Autodesk Inventor part; units mm, degrees
(part 2 of 2)
sketch "Esboço25" plane through (-2.4, 91.8, 35) normal (0, 1, 0) x (1, 0, 0)
  line L0 (50.4433, 30.11) -> (47.6201, 28.48)
  line L1 (50.4433, 33.37) -> (50.4433, 30.11)
  line L2 (47.6201, 28.48) -> (44.7968, 30.11)
  line L3 (44.7968, 30.11) -> (44.7968, 33.37)
  line L4 (47.6201, 35) -> (50.4433, 33.37)
  line L5 (44.7968, 33.37) -> (47.6201, 35)
  line L6 (47.6201, 28.48) -> (47.6201, 27.48)
  line L7 (50.4433, 22.59) -> (47.6201, 20.96)
  line L8 (50.4433, 25.85) -> (50.4433, 22.59)
  line L9 (47.6201, 20.96) -> (44.7968, 22.59)
  line L10 (44.7968, 22.59) -> (44.7968, 25.85)
  line L11 (47.6201, 27.48) -> (50.4433, 25.85)
  line L12 (44.7968, 25.85) -> (47.6201, 27.48)
  line L13 (47.6201, 20.96) -> (47.6201, 19.96)
  line L14 (50.4433, 15.07) -> (47.6201, 13.44)
  line L15 (50.4433, 18.33) -> (50.4433, 15.07)
  line L16 (47.6201, 13.44) -> (44.7968, 15.07)
  line L17 (44.7968, 15.07) -> (44.7968, 18.33)
  line L18 (47.6201, 19.96) -> (50.4433, 18.33)
  line L19 (44.7968, 18.33) -> (47.6201, 19.96)
  line L20 (47.6201, 13.44) -> (47.6201, 12.44)
  line L21 (50.4433, 7.55) -> (47.6201, 5.92)
  line L22 (50.4433, 10.81) -> (50.4433, 7.55)
  line L23 (47.6201, 5.92) -> (44.7968, 7.55)
  line L24 (44.7968, 7.55) -> (44.7968, 10.81)
  line L25 (47.6201, 12.44) -> (50.4433, 10.81)
  line L26 (44.7968, 10.81) -> (47.6201, 12.44)
  line L27 (47.6201, 5.92) -> (47.6201, 4.92)
  line L28 (47.6201, 1) -> (47.6201, 4.92)
  line L29 (47.6201, 1) -> (45.9227, 1.98)
  line L30 (45.9227, 1.98) -> (45.9227, 3.94)
  line L31 (45.9227, 3.94) -> (47.6201, 4.92)
  line L32 (47.6201, 4.92) -> (49.3175, 3.94)
  line L33 (49.3175, 3.94) -> (49.3175, 1.98)
  line L34 (49.3175, 1.98) -> (47.6201, 1)
  line L35 (39.9968, 30.11) -> (37.1736, 28.48)
  line L36 (39.9968, 33.37) -> (39.9968, 30.11)
  line L37 (37.1736, 28.48) -> (34.3504, 30.11)
  line L38 (34.3504, 30.11) -> (34.3504, 33.37)
  line L39 (37.1736, 35) -> (39.9968, 33.37)
  line L40 (34.3504, 33.37) -> (37.1736, 35)
  line L41 (37.1736, 28.48) -> (37.1736, 27.48)
  line L42 (37.1736, 20.96) -> (37.1736, 19.96)
  line L43 (39.9968, 22.59) -> (37.1736, 20.96)
  line L44 (37.1736, 20.96) -> (34.3504, 22.59)
  line L45 (39.9968, 25.85) -> (39.9968, 22.59)
  line L46 (34.3504, 22.59) -> (34.3504, 25.85)
  line L47 (37.1736, 27.48) -> (39.9968, 25.85)
  line L48 (34.3504, 25.85) -> (37.1736, 27.48)
  line L49 (37.1736, 13.44) -> (37.1736, 12.44)
  line L50 (39.9968, 15.07) -> (37.1736, 13.44)
  line L51 (37.1736, 13.44) -> (34.3504, 15.07)
  line L52 (39.9968, 18.33) -> (39.9968, 15.07)
  line L53 (34.3504, 15.07) -> (34.3504, 18.33)
  line L54 (37.1736, 19.96) -> (39.9968, 18.33)
  line L55 (34.3504, 18.33) -> (37.1736, 19.96)
  line L56 (37.1736, 5.92) -> (37.1736, 4.92)
  line L57 (39.9968, 7.55) -> (37.1736, 5.92)
  line L58 (37.1736, 5.92) -> (34.3504, 7.55)
  line L59 (39.9968, 10.81) -> (39.9968, 7.55)
  line L60 (34.3504, 7.55) -> (34.3504, 10.81)
  line L61 (37.1736, 12.44) -> (39.9968, 10.81)
  line L62 (34.3504, 10.81) -> (37.1736, 12.44)
  line L63 (37.1736, 1) -> (37.1736, 4.92)
  line L64 (37.1736, 1) -> (35.4762, 1.98)
  line L65 (35.4762, 1.98) -> (35.4762, 3.94)
  line L66 (35.4762, 3.94) -> (37.1736, 4.92)
  line L67 (37.1736, 4.92) -> (38.871, 3.94)
  line L68 (38.871, 3.94) -> (38.871, 1.98)
  line L69 (38.871, 1.98) -> (37.1736, 1)
  line L70 (29.5504, 30.11) -> (26.7271, 28.48)
  line L71 (29.5504, 33.37) -> (29.5504, 30.11)
  line L72 (26.7271, 28.48) -> (23.9039, 30.11)
  line L73 (23.9039, 30.11) -> (23.9039, 33.37)
  line L74 (26.7271, 35) -> (29.5504, 33.37)
  line L75 (23.9039, 33.37) -> (26.7271, 35)
  line L76 (26.7271, 28.48) -> (26.7271, 27.48)
  line L77 (26.7271, 20.96) -> (26.7271, 19.96)
  line L78 (29.5504, 22.59) -> (26.7271, 20.96)
  line L79 (26.7271, 20.96) -> (23.9039, 22.59)
  line L80 (29.5504, 25.85) -> (29.5504, 22.59)
  line L81 (23.9039, 22.59) -> (23.9039, 25.85)
  line L82 (26.7271, 27.48) -> (29.5504, 25.85)
  line L83 (23.9039, 25.85) -> (26.7271, 27.48)
  line L84 (26.7271, 13.44) -> (26.7271, 12.44)
  line L85 (29.5504, 15.07) -> (26.7271, 13.44)
  line L86 (26.7271, 13.44) -> (23.9039, 15.07)
  line L87 (29.5504, 18.33) -> (29.5504, 15.07)
  line L88 (23.9039, 15.07) -> (23.9039, 18.33)
  line L89 (26.7271, 19.96) -> (29.5504, 18.33)
  line L90 (23.9039, 18.33) -> (26.7271, 19.96)
  line L91 (26.8228, 5.92) -> (26.8228, 4.7542)
  line L92 (29.5504, 7.55) -> (26.7271, 5.92)
  line L93 (26.7271, 5.92) -> (23.9039, 7.55)
  line L94 (29.5504, 10.81) -> (29.5504, 7.55)
  line L95 (23.9039, 7.55) -> (23.9039, 10.81)
  line L96 (26.7271, 12.44) -> (29.5504, 10.81)
  line L97 (23.9039, 10.81) -> (26.7271, 12.44)
  line L98 (26.8228, 1.0553) -> (26.8228, 4.7542)
  line L99 (26.8228, 1.0553) -> (25.2211, 1.98)
  line L100 (25.2211, 1.98) -> (25.2211, 3.8295)
  line L101 (25.2211, 3.8295) -> (26.8228, 4.7542)
  line L102 (26.8228, 4.7542) -> (28.4245, 3.8295)
  line L103 (28.4245, 3.8295) -> (28.4245, 1.98)
  line L104 (28.4245, 1.98) -> (26.8228, 1.0553)
  line L105 (19.1039, 30.11) -> (16.2806, 28.48)
  line L106 (19.1039, 33.37) -> (19.1039, 30.11)
  line L107 (16.2806, 28.48) -> (13.4574, 30.11)
  line L108 (13.4574, 30.11) -> (13.4574, 33.37)
  line L109 (16.2806, 35) -> (19.1039, 33.37)
  line L110 (13.4574, 33.37) -> (16.2806, 35)
  line L111 (16.2806, 28.48) -> (16.2806, 27.48)
  line L112 (16.2806, 20.96) -> (16.2806, 19.96)
  line L113 (19.1039, 22.59) -> (16.2806, 20.96)
  line L114 (16.2806, 20.96) -> (13.4574, 22.59)
  line L115 (19.1039, 25.85) -> (19.1039, 22.59)
  line L116 (13.4574, 22.59) -> (13.4574, 25.85)
  line L117 (16.2806, 27.48) -> (19.1039, 25.85)
  line L118 (13.4574, 25.85) -> (16.2806, 27.48)
  line L119 (16.2806, 13.44) -> (16.2806, 12.44)
  line L120 (19.1039, 15.07) -> (16.2806, 13.44)
  line L121 (16.2806, 13.44) -> (13.4574, 15.07)
  line L122 (19.1039, 18.33) -> (19.1039, 15.07)
  line L123 (13.4574, 15.07) -> (13.4574, 18.33)
  line L124 (16.2806, 19.96) -> (19.1039, 18.33)
  line L125 (13.4574, 18.33) -> (16.2806, 19.96)
  line L126 (16.2806, 5.92) -> (16.2806, 4.92)
  line L127 (19.1039, 7.55) -> (16.2806, 5.92)
  line L128 (16.2806, 5.92) -> (13.4574, 7.55)
  line L129 (19.1039, 10.81) -> (19.1039, 7.55)
  line L130 (13.4574, 7.55) -> (13.4574, 10.81)
  line L131 (16.2806, 12.44) -> (19.1039, 10.81)
  line L132 (13.4574, 10.81) -> (16.2806, 12.44)
  line L133 (16.2806, 1) -> (16.2806, 4.92)
  line L134 (16.2806, 1) -> (14.5832, 1.98)
  line L135 (14.5832, 1.98) -> (14.5832, 3.94)
  line L136 (14.5832, 3.94) -> (16.2806, 4.92)
  line L137 (16.2806, 4.92) -> (17.978, 3.94)
  line L138 (17.978, 3.94) -> (17.978, 1.98)
  line L139 (17.978, 1.98) -> (16.2806, 1)
  line L140 (8.6574, 30.11) -> (5.8342, 28.48)
  line L141 (8.6574, 33.37) -> (8.6574, 30.11)
  line L142 (5.8342, 28.48) -> (3.0109, 30.11)
  line L143 (3.0109, 30.11) -> (3.0109, 33.37)
  line L144 (5.8342, 35) -> (8.6574, 33.37)
  line L145 (3.0109, 33.37) -> (5.8342, 35)
  line L146 (5.8342, 28.48) -> (5.8342, 27.48)
  line L147 (5.8342, 20.96) -> (5.8342, 19.96)
  line L148 (8.6574, 22.59) -> (5.8342, 20.96)
  line L149 (5.8342, 20.96) -> (3.0109, 22.59)
  line L150 (8.6574, 25.85) -> (8.6574, 22.59)
  line L151 (3.0109, 22.59) -> (3.0109, 25.85)
  line L152 (5.8342, 27.48) -> (8.6574, 25.85)
  line L153 (3.0109, 25.85) -> (5.8342, 27.48)
  line L154 (5.8342, 13.44) -> (5.8342, 12.44)
  line L155 (8.6574, 15.07) -> (5.8342, 13.44)
  line L156 (5.8342, 13.44) -> (3.0109, 15.07)
  line L157 (8.6574, 18.33) -> (8.6574, 15.07)
  line L158 (3.0109, 15.07) -> (3.0109, 18.33)
  line L159 (5.8342, 19.96) -> (8.6574, 18.33)
  line L160 (3.0109, 18.33) -> (5.8342, 19.96)
  line L161 (5.8769, 5.92) -> (5.8769, 4.8459)
  line L162 (8.6574, 7.55) -> (5.8342, 5.92)
  line L163 (5.8342, 5.92) -> (3.0109, 7.55)
  line L164 (8.6574, 10.81) -> (8.6574, 7.55)
  line L165 (3.0109, 7.55) -> (3.0109, 10.81)
  line L166 (5.8342, 12.44) -> (8.6574, 10.81)
  line L167 (3.0109, 10.81) -> (5.8342, 12.44)
  line L168 (5.8769, 1.0247) -> (5.8769, 4.8459)
  line L169 (5.8769, 1.0247) -> (4.2223, 1.98)
  line L170 (4.2223, 1.98) -> (4.2223, 3.8906)
  line L171 (4.2223, 3.8906) -> (5.8769, 4.8459)
  line L172 (5.8769, 4.8459) -> (7.5316, 3.8906)
  line L173 (7.5316, 3.8906) -> (7.5316, 1.98)
  line L174 (7.5316, 1.98) -> (5.8769, 1.0247)
  line L175 (3.0109, 9.18) -> (3.0109, 7.7242)
  line L176 (60.8898, 7.55) -> (58.0666, 5.92)
  line L177 (58.0666, 5.92) -> (55.2433, 7.55)
  line L178 (60.8898, 10.81) -> (60.8898, 7.55)
  line L179 (55.2433, 7.55) -> (55.2433, 10.81)
  line L180 (58.0666, 12.44) -> (60.8898, 10.81)
  line L181 (55.2433, 10.81) -> (58.0666, 12.44)
  line L182 (58.0666, 1) -> (56.3692, 1.98)
  line L183 (56.3692, 1.98) -> (56.3692, 3.94)
  line L184 (56.3692, 3.94) -> (58.0666, 4.92)
  line L185 (58.0666, 4.92) -> (59.764, 3.94)
  line L186 (59.764, 3.94) -> (59.764, 1.98)
  line L187 (59.764, 1.98) -> (58.0666, 1)
  line L188 (60.8898, 30.11) -> (58.0666, 28.48)
  line L189 (60.8898, 33.37) -> (60.8898, 30.11)
  line L190 (58.0666, 28.48) -> (55.2433, 30.11)
  line L191 (55.2433, 30.11) -> (55.2433, 33.37)
  line L192 (58.0666, 35) -> (60.8898, 33.37)
  line L193 (55.2433, 33.37) -> (58.0666, 35)
  line L194 (5.8342, 7.5447) -> (8.6574, 5.9147)
  line L195 (3.0109, 5.9147) -> (5.8342, 7.5447)
  line L196 (8.6574, 5.9147) -> (8.6574, 2.6547)
  line L197 (8.6574, 2.6547) -> (5.8342, 1.0247)
  line L198 (3.0109, 2.6547) -> (3.0109, 5.9147)
  line L199 (5.8342, 1.0247) -> (3.0109, 2.6547)
  line L200 (8.6574, 33.37) -> (8.6574, 2.6547)
  line L201 (3.0109, 33.37) -> (3.0109, 2.6547)
  line L202 (19.1039, 30.11) -> (16.2806, 28.48)
  line L203 (16.2806, 28.48) -> (13.4574, 30.11)
  line L204 (19.1039, 33.37) -> (19.1039, 30.11)
  line L205 (13.4574, 30.11) -> (13.4574, 33.37)
  line L206 (16.2806, 28.48) -> (16.2806, 27.48)
  line L207 (16.2806, 27.48) -> (19.1039, 25.85)
  line L208 (13.4574, 25.85) -> (16.2806, 27.48)
  line L209 (19.1039, 25.85) -> (19.1039, 22.59)
  line L210 (13.4574, 22.59) -> (13.4574, 25.85)
  line L211 (16.2806, 20.96) -> (13.4574, 22.59)
  line L212 (16.2806, 20.96) -> (16.2806, 19.96)
  line L213 (19.1039, 22.59) -> (16.2806, 20.96)
  line L214 (16.2806, 19.96) -> (19.1039, 18.33)
  line L215 (13.4574, 18.33) -> (16.2806, 19.96)
  line L216 (19.1039, 18.33) -> (19.1039, 15.07)
  line L217 (13.4574, 15.07) -> (13.4574, 18.33)
  line L218 (16.2806, 13.44) -> (13.4574, 15.07)
  line L219 (19.1039, 15.07) -> (16.2806, 13.44)
  line L220 (16.2806, 13.44) -> (16.2806, 12.44)
  line L221 (16.2806, 12.44) -> (19.1039, 10.81)
  line L222 (13.4574, 10.81) -> (16.2806, 12.44)
  line L223 (19.1039, 10.81) -> (19.1039, 7.55)
  line L224 (19.1039, 7.55) -> (16.2806, 5.92)
  line L225 (13.4574, 7.55) -> (13.4574, 10.81)
  line L226 (16.2806, 5.92) -> (13.4574, 7.55)
  line L227 (16.3234, 5.92) -> (16.3234, 4.8459)
  line L228 (14.6687, 3.8906) -> (16.3234, 4.8459)
  line L229 (16.3234, 4.8459) -> (17.978, 3.8906)
  line L230 (17.978, 3.8906) -> (17.978, 1.98)
  line L231 (14.6687, 1.98) -> (14.6687, 3.8906)
  line L232 (16.3234, 1.0247) -> (16.3234, 4.8459)
  line L233 (17.978, 1.98) -> (16.3234, 1.0247)
  line L234 (16.3234, 1.0247) -> (14.6687, 1.98)
  line L235 (16.2806, 35) -> (19.1039, 33.37)
  line L236 (13.4574, 33.37) -> (16.2806, 35)
  line L237 (13.4574, 9.18) -> (13.4574, 7.7242)
  line L238 (13.4574, 5.9147) -> (16.2806, 7.5447)
  line L239 (13.4574, 2.6547) -> (13.4574, 5.9147)
  line L240 (16.2806, 1.0247) -> (13.4574, 2.6547)
  line L241 (19.1039, 2.6547) -> (16.2806, 1.0247)
  line L242 (19.1039, 5.9147) -> (19.1039, 2.6547)
  line L243 (16.2806, 7.5447) -> (19.1039, 5.9147)
  line L244 (19.1039, 33.37) -> (19.1039, 2.6547)
  line L245 (13.4574, 33.37) -> (13.4574, 2.6547)
  line L246 (29.5504, 30.11) -> (26.7271, 28.48)
  line L247 (26.7271, 28.48) -> (23.9039, 30.11)
  line L248 (29.5504, 33.37) -> (29.5504, 30.11)
  line L249 (23.9039, 30.11) -> (23.9039, 33.37)
  line L250 (26.7271, 28.48) -> (26.7271, 27.48)
  line L251 (26.7271, 27.48) -> (29.5504, 25.85)
  line L252 (23.9039, 25.85) -> (26.7271, 27.48)
  line L253 (29.5504, 25.85) -> (29.5504, 22.59)
  line L254 (23.9039, 22.59) -> (23.9039, 25.85)
  line L255 (26.7271, 20.96) -> (23.9039, 22.59)
  line L256 (26.7271, 20.96) -> (26.7271, 19.96)
  line L257 (29.5504, 22.59) -> (26.7271, 20.96)
  line L258 (26.7271, 19.96) -> (29.5504, 18.33)
  line L259 (23.9039, 18.33) -> (26.7271, 19.96)
  line L260 (29.5504, 18.33) -> (29.5504, 15.07)
  line L261 (23.9039, 15.07) -> (23.9039, 18.33)
  line L262 (26.7271, 13.44) -> (23.9039, 15.07)
  line L263 (29.5504, 15.07) -> (26.7271, 13.44)
  line L264 (26.7271, 13.44) -> (26.7271, 12.44)
  line L265 (26.7271, 12.44) -> (29.5504, 10.81)
  line L266 (23.9039, 10.81) -> (26.7271, 12.44)
  line L267 (29.5504, 10.81) -> (29.5504, 7.55)
  line L268 (29.5504, 7.55) -> (26.7271, 5.92)
  line L269 (23.9039, 7.55) -> (23.9039, 10.81)
  line L270 (26.7271, 5.92) -> (23.9039, 7.55)
  line L271 (26.7699, 5.92) -> (26.7699, 4.8459)
  line L272 (25.1152, 3.8906) -> (26.7699, 4.8459)
  line L273 (26.7699, 4.8459) -> (28.4245, 3.8906)
  line L274 (28.4245, 3.8906) -> (28.4245, 1.98)
  line L275 (25.1152, 1.98) -> (25.1152, 3.8906)
  line L276 (26.7699, 1.0247) -> (26.7699, 4.8459)
  line L277 (28.4245, 1.98) -> (26.7699, 1.0247)
  line L278 (26.7699, 1.0247) -> (25.1152, 1.98)
  line L279 (26.7271, 35) -> (29.5504, 33.37)
  line L280 (23.9039, 33.37) -> (26.7271, 35)
  line L281 (23.9039, 9.18) -> (23.9039, 7.7242)
  line L282 (23.9039, 5.9147) -> (26.7271, 7.5447)
  line L283 (23.9039, 2.6547) -> (23.9039, 5.9147)
  line L284 (26.7271, 1.0247) -> (23.9039, 2.6547)
  line L285 (29.5504, 2.6547) -> (26.7271, 1.0247)
  line L286 (29.5504, 5.9147) -> (29.5504, 2.6547)
  line L287 (26.7271, 7.5447) -> (29.5504, 5.9147)
  line L288 (29.5504, 33.37) -> (29.5504, 2.6547)
  line L289 (23.9039, 33.37) -> (23.9039, 2.6547)
  line L290 (39.9968, 30.11) -> (37.1736, 28.48)
  line L291 (37.1736, 28.48) -> (34.3504, 30.11)
  line L292 (39.9968, 33.37) -> (39.9968, 30.11)
  line L293 (34.3504, 30.11) -> (34.3504, 33.37)
  line L294 (37.1736, 28.48) -> (37.1736, 27.48)
  line L295 (37.1736, 27.48) -> (39.9968, 25.85)
  line L296 (34.3504, 25.85) -> (37.1736, 27.48)
  line L297 (39.9968, 25.85) -> (39.9968, 22.59)
  line L298 (34.3504, 22.59) -> (34.3504, 25.85)
  line L299 (37.1736, 20.96) -> (34.3504, 22.59)
  line L300 (37.1736, 20.96) -> (37.1736, 19.96)
  line L301 (39.9968, 22.59) -> (37.1736, 20.96)
  line L302 (37.1736, 19.96) -> (39.9968, 18.33)
  line L303 (34.3504, 18.33) -> (37.1736, 19.96)
  line L304 (39.9968, 18.33) -> (39.9968, 15.07)
  line L305 (34.3504, 15.07) -> (34.3504, 18.33)
  line L306 (37.1736, 13.44) -> (34.3504, 15.07)
  line L307 (39.9968, 15.07) -> (37.1736, 13.44)
  line L308 (37.1736, 13.44) -> (37.1736, 12.44)
  line L309 (37.1736, 12.44) -> (39.9968, 10.81)
  line L310 (34.3504, 10.81) -> (37.1736, 12.44)
  line L311 (39.9968, 10.81) -> (39.9968, 7.55)
  line L312 (39.9968, 7.55) -> (37.1736, 5.92)
  line L313 (34.3504, 7.55) -> (34.3504, 10.81)
  line L314 (37.1736, 5.92) -> (34.3504, 7.55)
  line L315 (37.2164, 5.92) -> (37.2164, 4.8459)
  line L316 (35.5617, 3.8906) -> (37.2164, 4.8459)
  line L317 (37.2164, 4.8459) -> (38.871, 3.8906)
  line L318 (38.871, 3.8906) -> (38.871, 1.98)
  line L319 (35.5617, 1.98) -> (35.5617, 3.8906)
  line L320 (37.2164, 1.0247) -> (37.2164, 4.8459)
  line L321 (38.871, 1.98) -> (37.2164, 1.0247)
  line L322 (37.2164, 1.0247) -> (35.5617, 1.98)
  line L323 (37.1736, 35) -> (39.9968, 33.37)
  line L324 (34.3504, 33.37) -> (37.1736, 35)
  line L325 (34.3504, 9.18) -> (34.3504, 7.7242)
  line L326 (34.3504, 5.9147) -> (37.1736, 7.5447)
  line L327 (34.3504, 2.6547) -> (34.3504, 5.9147)
  line L328 (37.1736, 1.0247) -> (34.3504, 2.6547)
  line L329 (39.9968, 2.6547) -> (37.1736, 1.0247)
  line L330 (39.9968, 5.9147) -> (39.9968, 2.6547)
  line L331 (37.1736, 7.5447) -> (39.9968, 5.9147)
  line L332 (39.9968, 33.37) -> (39.9968, 2.6547)
  line L333 (34.3504, 33.37) -> (34.3504, 2.6547)
  line L334 (50.4433, 30.11) -> (47.6201, 28.48)
  line L335 (47.6201, 28.48) -> (44.7968, 30.11)
  line L336 (50.4433, 33.37) -> (50.4433, 30.11)
  line L337 (44.7968, 30.11) -> (44.7968, 33.37)
  line L338 (47.6201, 28.48) -> (47.6201, 27.48)
  line L339 (47.6201, 27.48) -> (50.4433, 25.85)
  line L340 (44.7968, 25.85) -> (47.6201, 27.48)
  line L341 (50.4433, 25.85) -> (50.4433, 22.59)
  line L342 (44.7968, 22.59) -> (44.7968, 25.85)
  line L343 (47.6201, 20.96) -> (44.7968, 22.59)
  line L344 (47.6201, 20.96) -> (47.6201, 19.96)
  line L345 (50.4433, 22.59) -> (47.6201, 20.96)
  line L346 (47.6201, 19.96) -> (50.4433, 18.33)
  line L347 (44.7968, 18.33) -> (47.6201, 19.96)
  line L348 (50.4433, 18.33) -> (50.4433, 15.07)
  line L349 (44.7968, 15.07) -> (44.7968, 18.33)
  line L350 (47.6201, 13.44) -> (44.7968, 15.07)
  line L351 (50.4433, 15.07) -> (47.6201, 13.44)
  line L352 (47.6201, 13.44) -> (47.6201, 12.44)
  line L353 (47.6201, 12.44) -> (50.4433, 10.81)
  line L354 (44.7968, 10.81) -> (47.6201, 12.44)
  line L355 (50.4433, 10.81) -> (50.4433, 7.55)
  line L356 (50.4433, 7.55) -> (47.6201, 5.92)
  line L357 (44.7968, 7.55) -> (44.7968, 10.81)
  line L358 (47.6201, 5.92) -> (44.7968, 7.55)
  line L359 (47.6628, 5.92) -> (47.6628, 4.8459)
  line L360 (46.0082, 3.8906) -> (47.6628, 4.8459)
  line L361 (47.6628, 4.8459) -> (49.3175, 3.8906)
  line L362 (49.3175, 3.8906) -> (49.3175, 1.98)
  line L363 (46.0082, 1.98) -> (46.0082, 3.8906)
  line L364 (47.6628, 1.0247) -> (47.6628, 4.8459)
  line L365 (49.3175, 1.98) -> (47.6628, 1.0247)
  line L366 (47.6628, 1.0247) -> (46.0082, 1.98)
  line L367 (47.6201, 35) -> (50.4433, 33.37)
  line L368 (44.7968, 33.37) -> (47.6201, 35)
  line L369 (44.7968, 9.18) -> (44.7968, 7.7242)
  line L370 (44.7968, 5.9147) -> (47.6201, 7.5447)
  line L371 (44.7968, 2.6547) -> (44.7968, 5.9147)
  line L372 (47.6201, 1.0247) -> (44.7968, 2.6547)
  line L373 (50.4433, 2.6547) -> (47.6201, 1.0247)
  line L374 (50.4433, 5.9147) -> (50.4433, 2.6547)
  line L375 (47.6201, 7.5447) -> (50.4433, 5.9147)
  line L376 (50.4433, 33.37) -> (50.4433, 2.6547)
  line L377 (44.7968, 33.37) -> (44.7968, 2.6547)
  line L378 (55.2433, 5.89) -> (58.0666, 7.52)
  line L379 (58.0666, 1) -> (55.2433, 2.63)
  line L380 (55.2433, 2.63) -> (55.2433, 5.89)
  line L381 (60.8898, 2.63) -> (58.0666, 1)
  line L382 (60.8898, 5.89) -> (60.8898, 2.63)
  line L383 (58.0666, 7.52) -> (60.8898, 5.89)
  line L384 (55.2433, 10.81) -> (55.2433, 2.63)
  line L385 (60.8898, 10.81) -> (60.8898, 2.63)
  point P0 (2.4, 35)
  point P1 (47.6201, 31.74)
  point P2 (0, 0)
  point P3 (47.6201, 24.22)
  point P4 (47.6201, 16.7)
  point P5 (47.6201, 2.96)
  point P6 (37.1736, 31.74)
  point P7 (37.1736, 24.22)
  point P8 (37.1736, 16.7)
  point P9 (37.1736, 9.18)
  point P10 (37.1736, 2.96)
  point P11 (26.7271, 31.74)
  point P12 (26.7271, 24.22)
  point P13 (26.7271, 16.7)
  point P14 (26.7271, 9.18)
  point P15 (26.8228, 2.9047)
  point P16 (16.2806, 31.74)
  point P17 (16.2806, 24.22)
  point P18 (16.2806, 16.7)
  point P19 (16.2806, 9.18)
  point P20 (16.2806, 2.96)
  point P21 (5.8342, 31.74)
  point P22 (5.8342, 24.22)
  point P23 (5.8342, 16.7)
  point P24 (5.8342, 9.18)
  point P25 (5.8769, 2.9353)
  point P26 (58.0666, 2.96)
  point P27 (58.0666, 31.74)
  point P28 (5.8342, 4.2847)
  point P29 (16.2806, 31.74)
  point P30 (16.2806, 24.22)
  point P31 (16.2806, 16.7)
  point P32 (16.2806, 9.18)
  point P33 (16.3234, 2.9353)
  point P34 (16.2806, 4.2847)
  point P35 (26.7271, 31.74)
  point P36 (26.7271, 24.22)
  point P37 (26.7271, 16.7)
  point P38 (26.7271, 9.18)
  point P39 (26.7699, 2.9353)
  point P40 (26.7271, 4.2847)
  point P41 (37.1736, 31.74)
  point P42 (37.1736, 24.22)
  point P43 (37.1736, 16.7)
  point P44 (37.1736, 9.18)
  point P45 (37.2164, 2.9353)
  point P46 (37.1736, 4.2847)
  point P47 (47.6201, 31.74)
  point P48 (47.6201, 24.22)
  point P49 (47.6201, 16.7)
  point P50 (47.6201, 9.18)
  point P51 (47.6628, 2.9353)
  point P52 (47.6201, 4.2847)
  point P53 (8.6574, 10.81)
  point P54 (3.0109, 10.81)
  point P55 (3.0109, 7.55)
  point P56 (3.0109, 5.9147)
  point P57 (5.8555, 1.037)
  point P58 (7.5316, 2.0047)
  point P59 (8.6574, 5.9147)
  point P60 (29.5504, 10.81)
  point P61 (26.7485, 1.037)
  point P62 (26.8228, 1.0553)
  point P63 (28.4245, 2.0047)
  point P64 (19.1039, 10.81)
  point P65 (19.1039, 7.55)
  point P66 (13.4574, 7.55)
  point P67 (14.5832, 2.0047)
  point P68 (17.978, 2.0047)
  point P69 (39.9968, 10.81)
  point P70 (34.3504, 10.81)
  point P71 (34.3504, 7.55)
  point P72 (35.4762, 2.0047)
  point P73 (38.871, 2.0047)
  point P74 (39.9968, 7.55)
  point P75 (50.4433, 10.81)
  point P76 (49.3175, 2.0047)
  point P77 (45.9227, 2.0047)
  point P78 (60.8898, 5.89)
  constraints: 772 end point, 51 vertical, 9 midpoint, 6 collinear, 5 point on line, 663 other
extrude "Extrusão17" cut sketch "Esboço25" against normal blind 10
sketch "Esboço26" plane through (0.2, -4.8, 15.5) normal (0, -1, 0) x (1, 0, 0)
  line L0 (0.4109, -13.8875) -> (0.4109, -10.6275)
  line L1 (0.4109, -10.6275) -> (3.2341, -8.9975)
  line L2 (3.2341, -15.5175) -> (0.4109, -13.8875)
  line L3 (3.2341, -8.9975) -> (6.0574, -10.6275)
  line L4 (6.0574, -10.6275) -> (6.0574, -13.8875)
  line L5 (6.0574, -13.8875) -> (3.2341, -15.5175)
  line L6 (10.824, -13.87) -> (10.824, -10.61)
  line L7 (10.824, -10.61) -> (13.6472, -8.98)
  line L8 (13.6472, -15.5) -> (10.824, -13.87)
  line L9 (13.6472, -8.98) -> (16.4705, -10.61)
  line L10 (16.4705, -10.61) -> (16.4705, -13.87)
  line L11 (16.4705, -13.87) -> (13.6472, -15.5)
  line L12 (21.2705, -13.87) -> (21.2705, -10.61)
  line L13 (21.2705, -10.61) -> (24.0937, -8.98)
  line L14 (24.0937, -15.5) -> (21.2705, -13.87)
  line L15 (24.0937, -8.98) -> (26.917, -10.61)
  line L16 (26.917, -10.61) -> (26.917, -13.87)
  line L17 (26.917, -13.87) -> (24.0937, -15.5)
  line L18 (31.717, -13.87) -> (31.717, -10.61)
  line L19 (31.717, -10.61) -> (34.5402, -8.98)
  line L20 (34.5402, -15.5) -> (31.717, -13.87)
  line L21 (34.5402, -8.98) -> (37.3634, -10.61)
  line L22 (37.3634, -10.61) -> (37.3634, -13.87)
  line L23 (37.3634, -13.87) -> (34.5402, -15.5)
  line L24 (42.1634, -13.87) -> (42.1634, -10.61)
  line L25 (42.1634, -10.61) -> (44.9867, -8.98)
  line L26 (44.9867, -15.5) -> (42.1634, -13.87)
  line L27 (44.9867, -8.98) -> (47.8099, -10.61)
  line L28 (47.8099, -10.61) -> (47.8099, -13.87)
  line L29 (47.8099, -13.87) -> (44.9867, -15.5)
  line L30 (52.6099, -13.87) -> (52.6099, -10.61)
  line L31 (52.6099, -10.61) -> (55.4332, -8.98)
  line L32 (55.4332, -15.5) -> (52.6099, -13.87)
  line L33 (55.4332, -8.98) -> (58.2564, -10.61)
  line L34 (58.2564, -10.61) -> (58.2564, -13.87)
  line L35 (58.2564, -13.87) -> (55.4332, -15.5)
  line L36 (0.4008, -6.35) -> (0.4109, -3.09)
  line L37 (0.4109, -3.09) -> (3.2392, -1.4687)
  line L38 (3.219, -7.9887) -> (0.4008, -6.35)
  line L39 (3.2392, -1.4687) -> (6.0574, -3.1075)
  line L40 (6.0574, -3.1075) -> (6.0473, -6.3675)
  line L41 (6.0473, -6.3675) -> (3.219, -7.9887)
  line L42 (10.824, -6.35) -> (10.824, -3.09)
  line L43 (10.824, -3.09) -> (13.6472, -1.46)
  line L44 (13.6472, -7.98) -> (10.824, -6.35)
  line L45 (13.6472, -1.46) -> (16.4705, -3.09)
  line L46 (16.4705, -3.09) -> (16.4705, -6.35)
  line L47 (16.4705, -6.35) -> (13.6472, -7.98)
  line L48 (21.2705, -6.35) -> (21.2705, -3.09)
  line L49 (21.2705, -3.09) -> (24.0937, -1.46)
  line L50 (24.0937, -7.98) -> (21.2705, -6.35)
  line L51 (24.0937, -1.46) -> (26.917, -3.09)
  line L52 (26.917, -3.09) -> (26.917, -6.35)
  line L53 (26.917, -6.35) -> (24.0937, -7.98)
  line L54 (31.717, -6.35) -> (31.717, -3.09)
  line L55 (31.717, -3.09) -> (34.5402, -1.46)
  line L56 (34.5402, -7.98) -> (31.717, -6.35)
  line L57 (34.5402, -1.46) -> (37.3634, -3.09)
  line L58 (37.3634, -3.09) -> (37.3634, -6.35)
  line L59 (37.3634, -6.35) -> (34.5402, -7.98)
  line L60 (42.1634, -6.35) -> (42.1634, -3.09)
  line L61 (42.1634, -3.09) -> (44.9867, -1.46)
  line L62 (44.9867, -7.98) -> (42.1634, -6.35)
  line L63 (44.9867, -1.46) -> (47.8099, -3.09)
  line L64 (47.8099, -3.09) -> (47.8099, -6.35)
  line L65 (47.8099, -6.35) -> (44.9867, -7.98)
  line L66 (52.6099, -6.35) -> (52.6099, -3.09)
  line L67 (52.6099, -3.09) -> (55.4332, -1.46)
  line L68 (55.4332, -7.98) -> (52.6099, -6.35)
  line L69 (55.4332, -1.46) -> (58.2564, -3.09)
  line L70 (58.2564, -3.09) -> (58.2564, -6.35)
  line L71 (58.2564, -6.35) -> (55.4332, -7.98)
  line L72 (6.0574, -3.1075) -> (6.0574, -13.8875)
  line L73 (0.4109, -3.09) -> (0.4109, -13.87)
  line L74 (10.8187, -13.8875) -> (10.8187, -10.6275)
  line L75 (10.8187, -10.6275) -> (13.642, -8.9975)
  line L76 (13.642, -15.5175) -> (10.8187, -13.8875)
  line L77 (13.642, -8.9975) -> (16.4652, -10.6275)
  line L78 (16.4652, -10.6275) -> (16.4652, -13.8875)
  line L79 (16.4652, -13.8875) -> (13.642, -15.5175)
  line L80 (10.8086, -6.35) -> (10.8187, -3.09)
  line L81 (10.8187, -3.09) -> (13.647, -1.4687)
  line L82 (13.6268, -7.9887) -> (10.8086, -6.35)
  line L83 (16.4551, -6.3675) -> (13.6268, -7.9887)
  line L84 (13.647, -1.4687) -> (16.4652, -3.1075)
  line L85 (16.4652, -3.1075) -> (16.4551, -6.3675)
  line L86 (16.4652, -3.1075) -> (16.4652, -13.8875)
  line L87 (10.8187, -3.09) -> (10.8187, -13.87)
  line L88 (21.2654, -13.8875) -> (21.2654, -10.6275)
  line L89 (21.2654, -10.6275) -> (24.0886, -8.9975)
  line L90 (24.0886, -15.5175) -> (21.2654, -13.8875)
  line L91 (24.0886, -8.9975) -> (26.9119, -10.6275)
  line L92 (26.9119, -10.6275) -> (26.9119, -13.8875)
  line L93 (26.9119, -13.8875) -> (24.0886, -15.5175)
  line L94 (21.2553, -6.35) -> (21.2654, -3.09)
  line L95 (21.2654, -3.09) -> (24.0937, -1.4687)
  line L96 (24.0735, -7.9887) -> (21.2553, -6.35)
  line L97 (26.9018, -6.3675) -> (24.0735, -7.9887)
  line L98 (24.0937, -1.4687) -> (26.9119, -3.1075)
  line L99 (26.9119, -3.1075) -> (26.9018, -6.3675)
  line L100 (26.9119, -3.1075) -> (26.9119, -13.8875)
  line L101 (21.2654, -3.09) -> (21.2654, -13.87)
  line L102 (31.7119, -13.8875) -> (31.7119, -10.6275)
  line L103 (31.7119, -10.6275) -> (34.5351, -8.9975)
  line L104 (34.5351, -15.5175) -> (31.7119, -13.8875)
  line L105 (34.5351, -8.9975) -> (37.3584, -10.6275)
  line L106 (37.3584, -10.6275) -> (37.3584, -13.8875)
  line L107 (37.3584, -13.8875) -> (34.5351, -15.5175)
  line L108 (31.7018, -6.35) -> (31.7119, -3.09)
  line L109 (31.7119, -3.09) -> (34.5402, -1.4687)
  line L110 (34.52, -7.9887) -> (31.7018, -6.35)
  line L111 (37.3483, -6.3675) -> (34.52, -7.9887)
  line L112 (34.5402, -1.4687) -> (37.3584, -3.1075)
  line L113 (37.3584, -3.1075) -> (37.3483, -6.3675)
  line L114 (37.3584, -3.1075) -> (37.3584, -13.8875)
  line L115 (31.7119, -3.09) -> (31.7119, -13.87)
  line L116 (42.1584, -13.8875) -> (42.1584, -10.6275)
  line L117 (42.1584, -10.6275) -> (44.9816, -8.9975)
  line L118 (44.9816, -15.5175) -> (42.1584, -13.8875)
  line L119 (44.9816, -8.9975) -> (47.8049, -10.6275)
  line L120 (47.8049, -10.6275) -> (47.8049, -13.8875)
  line L121 (47.8049, -13.8875) -> (44.9816, -15.5175)
  line L122 (42.1483, -6.35) -> (42.1584, -3.09)
  line L123 (42.1584, -3.09) -> (44.9867, -1.4687)
  line L124 (44.9665, -7.9887) -> (42.1483, -6.35)
  line L125 (47.7948, -6.3675) -> (44.9665, -7.9887)
  line L126 (44.9867, -1.4687) -> (47.8049, -3.1075)
  line L127 (47.8049, -3.1075) -> (47.7948, -6.3675)
  line L128 (47.8049, -3.1075) -> (47.8049, -13.8875)
  line L129 (42.1584, -3.09) -> (42.1584, -13.87)
  line L130 (52.6049, -13.8875) -> (52.6049, -10.6275)
  line L131 (52.6049, -10.6275) -> (55.4281, -8.9975)
  line L132 (55.4281, -15.5175) -> (52.6049, -13.8875)
  line L133 (55.4281, -8.9975) -> (58.2513, -10.6275)
  line L134 (58.2513, -10.6275) -> (58.2513, -13.8875)
  line L135 (58.2513, -13.8875) -> (55.4281, -15.5175)
  line L136 (52.5948, -6.35) -> (52.6049, -3.09)
  line L137 (52.6049, -3.09) -> (55.4332, -1.4687)
  line L138 (55.413, -7.9887) -> (52.5948, -6.35)
  line L139 (58.2412, -6.3675) -> (55.413, -7.9887)
  line L140 (55.4332, -1.4687) -> (58.2513, -3.1075)
  line L141 (58.2513, -3.1075) -> (58.2412, -6.3675)
  line L142 (58.2513, -3.1075) -> (58.2513, -13.8875)
  line L143 (52.6049, -3.09) -> (52.6049, -13.87)
  point P0 (0.4109, -6.3558)
  point P1 (0.4109, -10.6275)
  point P2 (11.5582, -2.6661)
  point P3 (10.8187, -6.3558)
  point P4 (10.8187, -10.6275)
  point P5 (16.4652, -13.873)
  point P6 (16.4652, -10.607)
  point P7 (16.4652, -6.353)
  point P8 (53.3163, -2.6822)
  point P9 (52.6049, -6.3558)
  point P10 (52.6049, -10.6275)
  point P11 (58.2513, -13.8729)
  point P12 (58.2513, -10.6071)
  point P13 (58.2513, -6.3529)
  point P14 (42.1584, -6.3558)
  point P15 (42.1584, -10.6275)
  point P16 (47.8049, -13.8729)
  point P17 (47.8049, -10.6071)
  point P18 (47.8049, -6.3529)
  point P19 (42.8698, -2.6822)
  point P20 (32.4234, -2.6822)
  point P21 (31.7119, -6.3558)
  point P22 (31.7119, -10.6275)
  point P23 (37.3584, -13.8729)
  point P24 (37.3584, -10.6071)
  point P25 (37.3584, -6.3529)
  point P26 (26.9119, -10.6071)
  point P27 (26.9119, -6.3529)
  point P28 (21.9769, -2.6822)
  point P29 (21.2654, -6.3558)
  point P30 (21.2654, -10.6275)
  point P31 (26.9119, -13.8729)
  constraints: 288 end point, 6 collinear, 6 vertical
extrude "Extrusão18" cut sketch "Esboço26" against normal blind 10
sketch "Esboço27" plane through (63.8, 10, 39.8) normal (1, 0, 0) x (0, 0, -1)
  line L0 (18.24, 56.3405) -> (19.87, 59.1637)
  line L1 (19.87, 59.1637) -> (23.13, 59.1637)
  line L2 (23.13, 59.1637) -> (24.76, 56.3405)
  line L3 (24.76, 56.3405) -> (23.13, 53.5173)
  line L4 (23.13, 53.5173) -> (19.87, 53.5173)
  line L5 (19.87, 53.5173) -> (18.24, 56.3405)
  line L6 (10.72, 56.3405) -> (12.35, 59.1637)
  line L7 (12.35, 59.1637) -> (15.61, 59.1637)
  line L8 (15.61, 59.1637) -> (17.24, 56.3405)
  line L9 (17.24, 56.3405) -> (15.61, 53.5173)
  line L10 (15.61, 53.5173) -> (12.35, 53.5173)
  line L11 (12.35, 53.5173) -> (10.72, 56.3405)
  line L12 (3.2, 56.3405) -> (4.83, 59.1637)
  line L13 (4.83, 59.1637) -> (8.09, 59.1637)
  line L14 (8.09, 59.1637) -> (9.72, 56.3405)
  line L15 (9.72, 56.3405) -> (8.09, 53.5173)
  line L16 (8.09, 53.5173) -> (4.83, 53.5173)
  line L17 (4.83, 53.5173) -> (3.2, 56.3405)
  line L18 (4.83, 59.1637) -> (23.13, 59.1637)
  line L19 (4.83, 53.5173) -> (23.13, 53.5173)
  line L20 (15.61, 12.3838) -> (17.24, 9.5605)
  line L21 (17.24, 9.5605) -> (15.61, 6.7373)
  line L22 (18.24, 9.5605) -> (19.87, 12.3838)
  line L23 (19.87, 6.7373) -> (18.24, 9.5605)
  line L24 (19.87, 12.3838) -> (23.13, 12.3838)
  line L25 (23.13, 6.7373) -> (19.87, 6.7373)
  line L26 (23.13, 12.3838) -> (24.76, 9.5605)
  line L27 (24.76, 9.5605) -> (23.13, 6.7373)
  line L28 (4.83, 6.7373) -> (3.2, 9.5605)
  line L29 (3.2, 9.5605) -> (4.83, 12.3838)
  line L30 (15.61, 6.7373) -> (12.35, 6.7373)
  line L31 (12.35, 12.3838) -> (15.61, 12.3838)
  line L32 (4.83, 6.7373) -> (23.13, 6.7373)
  line L33 (4.83, 12.3838) -> (23.13, 12.3838)
  line L34 (10.72, 9.5605) -> (12.35, 12.3838)
  line L35 (12.35, 6.7373) -> (10.72, 9.5605)
  line L36 (8.09, 12.3838) -> (9.72, 9.5605)
  line L37 (9.72, 9.5605) -> (8.09, 6.7373)
  line L38 (8.09, 6.7373) -> (4.83, 6.7373)
  line L39 (4.83, 12.3838) -> (8.09, 12.3838)
  line L40 (34.91, 1.9373) -> (38.17, 1.9373)
  line L41 (38.17, -3.7092) -> (34.91, -3.7092)
  line L42 (39.8, -0.8859) -> (38.17, -3.7092)
  line L43 (38.17, 1.9373) -> (39.8, -0.8859)
  line L44 (33.28, -0.8859) -> (34.91, 1.9373)
  line L45 (34.91, -3.7092) -> (33.28, -0.8859)
  line L46 (30.65, 1.9373) -> (32.28, -0.8859)
  line L47 (32.28, -0.8859) -> (30.65, -3.7092)
  line L48 (27.39, 1.9373) -> (30.65, 1.9373)
  line L49 (30.65, -3.7092) -> (27.39, -3.7092)
  line L50 (27.39, -3.7092) -> (25.76, -0.8859)
  line L51 (25.76, -0.8859) -> (27.39, 1.9373)
  line L52 (38.17, 1.9373) -> (27.39, 1.9373)
  line L53 (38.17, -3.7092) -> (27.39, -3.7092)
  point P0 (21.5, 56.3405)
  point P1 (13.98, 56.3405)
  point P2 (6.46, 56.3405)
  point P3 (12.35, 53.5173)
  point P4 (15.61, 53.5173)
  point P5 (19.87, 53.5173)
  point P6 (19.87, 59.1637)
  point P7 (15.61, 59.1637)
  point P8 (12.35, 59.1637)
  point P9 (21.5, 9.5605)
  point P10 (13.98, 9.5605)
  point P11 (6.46, 9.5605)
  point P12 (12.35, 6.7373)
  point P13 (15.61, 6.7373)
  point P14 (36.54, -0.8859)
  point P15 (29.02, -0.8859)
  constraints: 108 end point, 4 collinear, 1 horizontal, 1 parallel, 104 other
extrude "Extrusão19" cut sketch "Esboço27" against normal blind 10
sketch "Esboço28" plane through (0, 0, -2.4) normal (0, 0, -1) x (-1, 0, 0)
  line L0 (4.8, 91.8) -> (-61.3, 91.8) projected
  line L1 (-63.8, 10) -> (-63.8, 91.8) projected
  line L2 (4.8, 91.8) -> (-63.8, 91.8)
  line L3 (-29.5, 91.8) -> (-29.5, -4.8)
  line L4 (-58.8, -4.8) -> (-0.2, -4.8) projected
  line L5 (-29.5, 43.5) -> (-63.8, 43.5)
  line L6 (-29.5, 43.5) -> (4.8, 43.5)
  line L7 (-29.5, 43.5) -> (4.8, 43.5) construction
  line L8 (-63.8, 43.5) -> (-53.8, 43.5)
  line L9 (4.8, 43.5) -> (-5.2, 43.5)
  line L10 (-29.5, -4.8) -> (-29.5, 5.2)
  line L11 (-29.5, 91.8) -> (-29.5, 81.8)
  line L12 (-29.5, 5.2) -> (-5.2, 5.2)
  line L13 (-5.2, 5.2) -> (-5.2, 43.5)
  line L14 (-29.5, 81.8) -> (-5.2, 81.8)
  line L15 (-5.2, 81.8) -> (-5.2, 43.5)
  line L16 (-29.5, 81.8) -> (-53.8, 81.8)
  line L17 (-53.8, 81.8) -> (-53.8, 43.5)
  line L18 (-29.5, 5.2) -> (-53.8, 5.2)
  line L19 (-53.8, 5.2) -> (-53.8, 43.5)
  point P0 (0, 0)
  dimension "d245" = 10
  dimension "d246" = 10
  dimension "d247" = 10
  dimension "d248" = 10
  constraints: 34 end point, 9 point on line, 7 perpendicular, 3 midpoint, 1 collinear, 1 horizontal, 1 parallel
  measures "d245" distance of L5.end L8.end
  measures "d246" distance of L7.end L9.end
  measures "d247" distance of L3.end L10.end
  measures "d248" distance of L3.start L11.end
extrude "Extrusão20" cut sketch "Esboço28" against normal blind 10 contours L14 L15 L6 L3 | L3 L5 L17 L16 | L6 L13 L12 L3 | L3 L18 L19 L5
fillet "Arredondamento4" radius 10 4 edges at (5.2, 5.2, -1.2) (53.8, 5.2, -1.2) (53.8, 81.8, -1.2) (5.2, 81.8, -1.2)
sketch "Esboço29" plane through (61.3, -4.8, -2.4) normal (1, 0, 0) x (0, 0, -1)
  line L0 (-11.4, 94.1) -> (-18.9, 94.1) projected
  line L1 (-15.2, 66.3) -> (-15.2, 75.981) projected
  line L2 (-18.9, 94.1) -> (-11.4, 94.1)
  line L3 (-12.7, 75.981) -> (-32.8, 75.981) projected
  line L4 (-19.6037, 75.981) -> (-11.0667, 75.981)
  line L5 (-15.15, 94.1) -> (-15.15, 75.981)
  circle A0 centre (-15.15, 85.0405) radius 1.45
  point P0 (-2.4, 4.8)
  dimension "d252" = 2.9
  constraints: 6 end point, 2 midpoint, 2 point on line, 1 centre point, 1 collinear, 1 horizontal, 1 perpendicular
  measures "d252" diameter of A0
extrude "Extrusão21" cut sketch "Esboço29" against normal blind 10
sketch "Esboço30" plane through (63.8, 10, 39.8) normal (1, 0, 0) x (0, 0, -1)
  line L0 (3.2, 9.5605) -> (4.8, 6.7893) projected
  line L1 (0.5, 0) -> (0.5, 81.8) projected
  line L2 (4.8, 0) -> (4.8, 6.7893) projected
  arc A0 (2.4, 4.8946) -> (2.4, 1.8946) centre (2.4, 3.3946) ccw
  line L3 (2.4, 0) -> (2.4, 81.8) projected
  line L4 (2.4, 3.3946) -> (2.4, 0)
  line L5 (2.4, 0) -> (2.4, 6.7893)
  point P0 (39.8, -10)
  point P1 (0, 0)
  point P2 (2.4, 1.8946)
  point P3 (2.4, 4.8946)
  dimension "d267" = 3
  constraints: 4 end point, 3 point on line, 2 point on circle, 1 centre point, 1 collinear
  measures "d267" diameter of A0
revolve "Revolução1" cut sketch "Esboço30" angle 360 about axis through (63.8, 10, 37.4) along (0, 1, 0)
sketch "Esboço31" plane through (-4.8, 91.8, -2.4) normal (-1, 0, 0) x (0, 0, 1)
  arc A0 (39.8, -79.9054) -> (39.8, -76.9054) centre (39.8, -78.4054) ccw
  line L0 (39.8, -81.8) -> (39.8, -74.3224)
  line L1 (42.2, -81.8) -> (42.2, -75.0627)
  line L2 (37.37, -75.0627) -> (42.2, -75.0627)
  line L3 (37.4, -81.8) -> (37.4, -75.0107) projected
  line L4 (37.4, -75.0107) -> (37.4, -81.8)
  line L5 (37.4, -81.8) -> (26.9, -81.8) projected
  line L6 (37.4, -81.8) -> (26.9, -81.8)
  line L7 (42.2, -81.8) -> (42.2, -96.6)
  line L8 (17.9, -91.6) -> (17.9, -96.6) projected
  line L9 (42.2, -96.6) -> (17.9, -96.6)
  line L10 (17.9, -96.6) -> (17.9, -90.8)
  arc A1 (26.9, -81.8) -> (17.9, -90.8) centre (26.9, -90.8) ccw projected
  arc A2 (26.9, -81.8) -> (17.9, -90.8) centre (26.9, -90.8) ccw
  point P0 (2.4, -91.8)
  constraints: 16 end point, 5 point on circle, 2 centre point, 2 perpendicular, 2 point on line, 2 vertical, 1 coincident, 1 collinear, 1 concentric
revolve "Revolução2" cut sketch "Esboço31" angle 360 about axis through (-4.8, 10, 37.4) along (0, 1, 0) contours L0 A0
sketch "Esboço33" plane through (0, 0, 15.5) normal (0, 0, 1) x (1, 0, 0)
  point P0 (0, 0)
